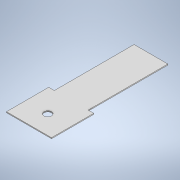
# Autodesk Inventor part: PendulumBackplate
Saved by Autodesk Inventor 2022.3 (Build 263350000, 350)
## iProperties
Created: 2023-10-29
Part Number: PendulumBackplate
Material: Generic
Document SubType Name: Modeling
Designer: Siggi
Density: 1 g/cm^3
Appearance: Default
Author: Siggi
Autodesk Inventor part; units mm, degrees
ref_plane "YZ Plane" through (0, 0, 0) normal (1, 0, 0) x (0, 1, 0)
ref_plane "XZ Plane" through (0, 0, 0) normal (0, 1, 0) x (-1, 0, 0)
ref_plane "XY Plane" through (0, 0, 0) normal (0, 0, 1) x (1, 0, 0)
sketch "Sketch1" plane through (0, 0, 0) normal (0, 1, 0) x (-1, 0, 0)
  line L0 (-48, 0) -> (-48, 45)
  line L1 (-48, 45) -> (0, 45)
  line L2 (0, 45) -> (0, 0)
  line L3 (-6, 0) -> (-6, -85)
  line L4 (-6, -85) -> (-42, -85)
  line L5 (-42, -85) -> (-42, 0)
  line L6 (-24, 45) -> (-24, 29)
  circle A0 centre (-24, 25) radius 4
  line L7 (0, 0) -> (-6, 0)
  line L8 (-42, 0) -> (-48, 0)
  dimension "d8" = 8
  dimension "d0" = 48
  dimension "d1" = 45
  dimension "d2" = 36
  dimension "d3" = 85
  dimension "d6" = 16
  dimension "d7" = 6
  constraints: 18 end point, 4 parallel, 2 horizontal, 2 perpendicular, 1 midpoint, 1 vertical, 1 vertical alignment, 2 other
  measures "d0" distance of L0.end L1.end
  measures "d1" distance of L0.start L0.end
  measures "d2" distance of L3.end L4.end
  measures "d3" distance of L3.start L3.end
  measures "d6" distance of L6.start L6.end
  measures "d7" distance of L5.end L0.start
extrude "Extrusion1" add sketch "Sketch1" along normal blind 1
body "Solid1"
